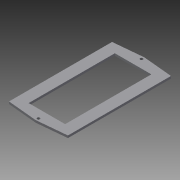
# Autodesk Inventor part: B layer cap
Saved by Autodesk Inventor 2014 SP1 (Build 180222100, 222)
## iProperties
Created: 2017-07-20
Part Number: B layer cap
Material: Generic
Document SubType Name: Modeling
Designer: kteo17
Density: 1 g/cm^3
Appearance: Default
Author: kteo17
Autodesk Inventor part; units mm, degrees
ref_plane "YZ Plane" through (0, 0, 0) normal (1, 0, 0) x (0, 1, 0)
ref_plane "XZ Plane" through (0, 0, 0) normal (0, 1, 0) x (-1, 0, 0)
ref_plane "XY Plane" through (0, 0, 0) normal (0, 0, 1) x (1, 0, 0)
sketch "Sketch1" plane through (0, 0, 0) normal (0, 0, 1) x (1, 0, 0)
  line L0 (66.675, 0) -> (66.675, 116.586)
  line L1 (0, 116.586) -> (0, 0)
  line L2 (12.7, 107.061) -> (53.975, 107.061)
  line L3 (53.975, 107.061) -> (53.975, 9.525)
  line L4 (53.975, 9.525) -> (12.7, 9.525)
  line L5 (12.7, 9.525) -> (12.7, 107.061)
  circle A0 centre (33.3375, 116.586) radius 1.5875
  circle A1 centre (33.3375, 0) radius 1.5875
  line L6 (0, 0) -> (33.3375, -3.175)
  line L7 (33.3375, -3.175) -> (66.675, 0)
  line L8 (0, 116.586) -> (33.3375, 119.761)
  line L9 (33.3375, 119.761) -> (66.675, 116.586)
  dimension "d2" = 12.7
  dimension "d5" = 66.675
  dimension "d6" = 116.586
  dimension "d9" = 9.525
  dimension "d12" = 9.525
  constraints: 20 end point, 5 parallel, 2 centre point, 1 perpendicular
  measures "d2" distance between parallel lines of L0 L3
  measures "d5" distance between parallel lines of L0 L1
  measures "d6" distance of L0.start L0.end
  measures "d9" distance from line of L4 A1.centre
  measures "d12" distance from line of L2 A0.centre
extrude "Extrusion1" add sketch "Sketch1" along normal blind 2.54
body "Solid1"
